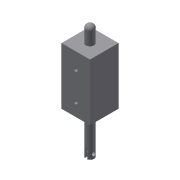
# Autodesk Inventor part: 00_springloaded_electromagnet
Saved by Autodesk Inventor 2019.4 (Build 234330000, 330)
## iProperties
Created: 2021-06-24
Part Number: 00_springloaded_electromagnet
Material: Generic
Document SubType Name: Modeling
Designer: diederichbenedict
Density: 1 g/cm^3
Appearance: Default
Author: diederichbenedict
Autodesk Inventor part; units mm, degrees
ref_plane "YZ Plane" through (0, 0, 0) normal (1, 0, 0) x (0, 1, 0)
ref_plane "XZ Plane" through (0, 0, 0) normal (0, 1, 0) x (-1, 0, 0)
ref_plane "XY Plane" through (0, 0, 0) normal (0, 0, 1) x (1, 0, 0)
sketch "Sketch1" plane through (0, 0, 0) normal (0, 1, 0) x (-1, 0, 0)
  line L0 (-7.6, -7.6) -> (7.6, -7.6)
  line L1 (7.6, -7.6) -> (7.6, 7.6)
  line L2 (7.6, 7.6) -> (-7.6, 7.6)
  line L3 (-7.6, 7.6) -> (-7.6, -7.6)
  line L4 (-7.6, -7.6) -> (7.6, 7.6) construction
  line L5 (7.6, -7.6) -> (-7.6, 7.6) construction
  point P0 (0, 0)
  dimension "d0" = 15.2
  dimension "d1" = 15.2
  constraints: 12 end point, 2 midpoint, 2 parallel, 1 horizontal, 1 perpendicular
  measures "d0" distance of L2.end L1.end
  measures "d1" distance of L1.end L0.end
extrude "Extrusion1" add sketch "Sketch1" along normal blind 30.3
sketch "Sketch2" plane through (0, 0, 0) normal (0, -1, 0) x (1, 0, 0)
  line L0 (7.6, -7.6) -> (-7.6, -7.6) projected
  line L1 (7.6, 7.6) -> (7.6, -7.6) projected
  line L2 (-7.6, 7.6) -> (7.6, 7.6) projected
  line L3 (-7.6, -7.6) -> (-7.6, 7.6) projected
  circle A0 centre (0, 0) radius 2.196
  constraints: 1 centre point, 1 coincident
extrude "Extrusion2" add sketch "Sketch2" along normal blind 22 contours A0
sketch "Sketch3" plane through (0, 30.3, 0) normal (0, 1, 0) x (1, 0, 0)
  circle A0 centre (0, 0) radius 2.196 projected
extrude "Extrusion3" add sketch "Sketch3" along normal blind 9
sketch "Sketch4" plane through (-7.6, 0, 7.6) normal (0, 0, 1) x (1, 0, 0)
  line L0 (0, 0) -> (15.2, 0) projected
  line L1 (15.2, 0) -> (15.2, 30.3) projected
  line L2 (0, 30.3) -> (15.2, 30.3) projected
  line L3 (0, 0) -> (0, 30.3) projected
  circle A0 centre (7.5, 21.8462) radius 1
  circle A1 centre (7.5, 6.8462) radius 1
  point P0 (7.6, 0)
  dimension "d8" = 2
  dimension "d9" = 2
  dimension "d10" = 15
  dimension "d11" = 0
  dimension "d12" = 7.5
  constraints: 2 centre point
  measures "d8" diameter of A0
  measures "d9" diameter of A1
  measures "d10" distance of A1.centre A0.centre
  measures "d11" horizontal distance of A0.centre A1.centre
  measures "d12" distance from line of A0.centre L3
extrude "Extrusion4" cut sketch "Sketch4" against normal blind 9 contours A0 | A1
fillet "Fillet1" radius 2 1 edges at (-2.196, 39.3, 0)
sketch "Sketch5" plane through (-7.6, 0, 7.6) normal (0, 0, 1) x (1, 0, 0)
  line L0 (5.404, -22) -> (9.796, -22) projected
  line L1 (9.796, 0) -> (5.404, 0) projected
  line L2 (6.9119, -26.9089) -> (8.2881, -26.9089)
  line L3 (8.2881, -26.9089) -> (8.2881, -17.0911)
  line L4 (8.2881, -17.0911) -> (6.9119, -17.0911)
  line L5 (6.9119, -17.0911) -> (6.9119, -26.9089)
  line L6 (5.404, -22) -> (9.796, -22) projected
  line L7 (6.9119, -26.9089) -> (8.2881, -17.0911) construction
  line L8 (8.2881, -26.9089) -> (6.9119, -17.0911) construction
  point P0 (7.6, 0)
  point P1 (7.6, -22)
  constraints: 12 end point, 3 midpoint, 2 parallel, 1 horizontal, 1 perpendicular
extrude "Extrusion5" cut sketch "Sketch5" against normal through all
sketch "Sketch6" plane through (-0.6881, -22, -2.0854) normal (1, 0, 0) x (0, 0, -1)
  line L0 (0, 4.9089) -> (0, 0) projected
  line L1 (-4.1707, 0) -> (0, 0) projected
  line L2 (-4.1707, 0) -> (-4.1707, 4.9089) projected
  line L3 (-4.1707, 4.9089) -> (-4.1707, 4.9089) projected
  line L4 (-4.1707, 4.9089) -> (-4.1707, 0) projected
  line L5 (0, 0) -> (-4.1707, 0) projected
  line L6 (0, 0) -> (0, 4.9089) projected
  line L7 (0, 4.9089) -> (0, 4.9089) projected
  line L8 (0.1106, 22) -> (-4.2813, 22) projected
  circle A0 centre (-2.0854, 2.269) radius 1
  point P0 (-2.0854, 22)
  dimension "d18" = 2
  constraints: 1 centre point
  measures "d18" diameter of A0
extrude "Extrusion6" cut sketch "Sketch6" along normal mid plane 9
ref_plane "Work Plane1" through (7.6, 0, 0) normal (0, 0, -1) x (-1, 0, 0)
sketch "Sketch7" plane through (7.6, 0, 0) normal (0, 0, -1) x (-1, 0, 0)
  circle A0 centre (11.376, -0.643) radius 0.5814
  point P0 (7.6, 0)
  constraints: 1 centre point
coil "Coil1" sketch "Sketch7" operation add axis through (0, 0, 0) along (0, -1, 0) pitch 5 turns 3 hand right
ref_plane "Work Plane2" through (0, -16.3411, 0) normal (0, -1, 0) x (1, 0, 0)
sketch "Sketch8" plane through (0, -16.3411, 0) normal (0, -1, 0) x (1, 0, 0)
  arc A0 (0.6881, -2.0854) -> (0.6881, 2.0854) centre (0, 0) ccw projected
  circle A1 centre (0, 0) radius 0.196 projected
  circle A2 centre (0, 0) radius 4.2328
  constraints: 1 centre point, 1 coincident
extrude "Extrusion7" add sketch "Sketch8" against normal blind 1
body "Solid1"
